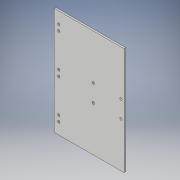
# Autodesk Inventor part: 11 deur plaat
Saved by Autodesk Inventor 2019 (Build 230136000, 136)
## iProperties
Created: 2021-01-22
Part Number: 11 deur plaat
Material: Generic
Document SubType Name: Sheet Metal
Designer: Stefan
Density: 1 g/cm^3
Sheet Metal Rule: Default_mm
Appearance: Default
Author: Stefan
Autodesk Inventor part; units mm, degrees
ref_plane "YZ Plane" through (0, 0, 0) normal (1, 0, 0) x (0, 1, 0)
ref_plane "XZ Plane" through (0, 0, 0) normal (0, 1, 0) x (-1, 0, 0)
ref_plane "XY Plane" through (0, 0, 0) normal (0, 0, 1) x (1, 0, 0)
sketch "Sketch1" plane through (0, 0, 0) normal (0, 0, 1) x (1, 0, 0)
  line L0 (-90.5, -90.5) -> (90.5, -90.5)
  line L1 (90.5, -90.5) -> (90.5, 90.5)
  line L2 (90.5, 90.5) -> (-90.5, 90.5)
  line L3 (-90.5, 90.5) -> (-90.5, -90.5)
  line L4 (-90.5, -90.5) -> (90.5, 90.5) construction
  line L5 (90.5, -90.5) -> (-90.5, 90.5) construction
  point P0 (0, 0)
  dimension "d0" = 181
  dimension "d1" = 181
  constraints: 12 end point, 2 midpoint, 2 parallel, 1 horizontal, 1 perpendicular
  measures "d0" distance of L2.end L1.end
  measures "d1" distance of L1.end L0.end
extrude "Extrusion1" add sketch "Sketch1" along normal blind 3
sketch "Sketch3" plane through (0, 0, 3) normal (0, 0, 1) x (1, 0, 0)
  line L0 (-90.5, 90.5) -> (-90.5, -90.5) projected
  line L1 (-90.5, 82.5) -> (-87.5, 82.5)
  line L2 (-87.5, 82.5) -> (-87.5, 67.5)
  line L3 (-87.5, 67.5) -> (-90.5, 67.5)
  line L4 (-90.5, 67.5) -> (-90.5, 82.5)
  line L5 (-85, 93.5) -> (-90.5, 93.5) projected
  line L6 (-90.5, 52.5) -> (-87.5, 52.5)
  line L7 (-87.5, 52.5) -> (-87.5, 37.5)
  line L8 (-87.5, 37.5) -> (-90.5, 37.5)
  line L9 (-90.5, 37.5) -> (-90.5, 52.5)
  line L10 (-90.5, 22.5) -> (-87.5, 22.5)
  line L11 (-87.5, 22.5) -> (-87.5, 7.5)
  line L12 (-87.5, 7.5) -> (-90.5, 7.5)
  line L13 (-90.5, 7.5) -> (-90.5, 22.5)
  line L14 (-90.5, -7.5) -> (-87.5, -7.5)
  line L15 (-87.5, -7.5) -> (-87.5, -22.5)
  line L16 (-87.5, -22.5) -> (-90.5, -22.5)
  line L17 (-90.5, -22.5) -> (-90.5, -7.5)
  line L18 (-90.5, -37.5) -> (-87.5, -37.5)
  line L19 (-87.5, -37.5) -> (-87.5, -52.5)
  line L20 (-87.5, -52.5) -> (-90.5, -52.5)
  line L21 (-90.5, -52.5) -> (-90.5, -37.5)
  line L22 (-90.5, -67.5) -> (-87.5, -67.5)
  line L23 (-87.5, -67.5) -> (-87.5, -82.5)
  line L24 (-87.5, -82.5) -> (-90.5, -82.5)
  line L25 (-90.5, -82.5) -> (-90.5, -67.5)
  line L26 (87.5, 82.5) -> (90.5, 82.5)
  line L27 (90.5, 82.5) -> (90.5, 67.5)
  line L28 (90.5, 67.5) -> (87.5, 67.5)
  line L29 (87.5, 67.5) -> (87.5, 82.5)
  line L30 (87.5, 52.5) -> (90.5, 52.5)
  line L31 (90.5, 52.5) -> (90.5, 37.5)
  line L32 (90.5, 37.5) -> (87.5, 37.5)
  line L33 (87.5, 37.5) -> (87.5, 52.5)
  line L34 (87.5, 22.5) -> (90.5, 22.5)
  line L35 (90.5, 22.5) -> (90.5, 7.5)
  line L36 (90.5, 7.5) -> (87.5, 7.5)
  line L37 (87.5, 7.5) -> (87.5, 22.5)
  line L38 (87.5, -7.5) -> (90.5, -7.5)
  line L39 (90.5, -7.5) -> (90.5, -22.5)
  line L40 (90.5, -22.5) -> (87.5, -22.5)
  line L41 (87.5, -22.5) -> (87.5, -7.5)
  line L42 (87.5, -37.5) -> (90.5, -37.5)
  line L43 (90.5, -37.5) -> (90.5, -52.5)
  line L44 (90.5, -52.5) -> (87.5, -52.5)
  line L45 (87.5, -52.5) -> (87.5, -37.5)
  line L46 (87.5, -67.5) -> (90.5, -67.5)
  line L47 (90.5, -67.5) -> (90.5, -82.5)
  line L48 (90.5, -82.5) -> (87.5, -82.5)
  line L49 (87.5, -82.5) -> (87.5, -67.5)
  point P0 (0, 0)
  point P1 (-90.5, -93.5)
  dimension "d27" = 3
  dimension "d28" = 15
  dimension "d29" = 11
  dimension "d32" = 30
  dimension "d35" = 178
  constraints: 96 end point, 2 horizontal, 2 parallel, 1 perpendicular, 1 point on line, 1 vertical, 88 other
  measures "d27" distance of L2.end L3.end
  measures "d28" distance of L1.end L2.end
  measures "d29" distance between parallel lines of L5 L1
  measures "d32" distance of L1.start L6.start
  measures "d35" distance of L1.start L26.start
extrude "Extrusion3" cut sketch "Sketch3" against normal blind 3
sketch "Sketch4" plane through (0, 0, 3) normal (0, 0, 1) x (1, 0, 0)
  line L0 (80, 93.5) -> (85.5, 93.5) projected
  line L1 (90.5, 90.5) -> (-90.5, 90.5) projected
  line L2 (85.5, 93.5) -> (90.5, 93.5)
  line L3 (90.5, 93.5) -> (90.5, 90.5)
  line L4 (90.5, 90.5) -> (85.5, 90.5)
  line L5 (85.5, 90.5) -> (85.5, 93.5)
  line L6 (-90.5, -90.5) -> (90.5, -90.5) projected
  line L7 (85.5, -90.5) -> (90.5, -90.5)
  line L8 (90.5, -90.5) -> (90.5, -93.5)
  line L9 (90.5, -93.5) -> (85.5, -93.5)
  line L10 (85.5, -93.5) -> (85.5, -90.5)
  point P0 (0, 0)
  point P1 (85.5, 90.5)
  dimension "d40" = 184
  constraints: 16 end point, 4 parallel, 2 horizontal, 2 perpendicular, 1 point on line
  measures "d40" distance between parallel lines of L1 L9
extrude "Extrusion4" add sketch "Sketch4" against normal blind 3
sketch "Sketch6" plane through (0, 0, 0) normal (0, 0, -1) x (-1, 0, 0)
  line L0 (-90.5, 82.5) -> (-90.5, 93.5) projected
  line L1 (-90.5, 93.5) -> (-75, 93.5)
  line L2 (-75, 93.5) -> (-75, -93.5)
  line L3 (-75, -93.5) -> (-90.5, -93.5)
  line L4 (-90.5, -93.5) -> (-90.5, 93.5)
  line L5 (85, 93.5) -> (90.5, 93.5) projected
  line L6 (90.5, 93.5) -> (46.5, 93.5)
  line L7 (46.5, 93.5) -> (46.5, -93.5)
  line L8 (46.5, -93.5) -> (90.5, -93.5)
  line L9 (90.5, -93.5) -> (90.5, 93.5)
  point P0 (0, 0)
  dimension "d47" = 15.5
  dimension "d48" = 44
  dimension "d49" = 187
  dimension "d50" = 187
  constraints: 16 end point, 4 parallel, 2 horizontal, 2 perpendicular
  measures "d47" distance of L2.end L3.end
  measures "d48" distance of L8.end L7.end
  measures "d49" distance between parallel lines of L5 L3
  measures "d50" distance between parallel lines of L8 L5
extrude "Extrusion6" cut sketch "Sketch6" against normal blind 10
sketch "Sketch7" plane through (0, 0, 3) normal (0, 0, 1) x (1, 0, 0)
  circle A0 centre (-38.5, 73.5) radius 2
  circle A1 centre (-38.5, 63.5) radius 2
  circle A2 centre (-38.5, 5) radius 2
  circle A3 centre (-38.5, -5) radius 2
  circle A4 centre (-38.5, -63.5) radius 2
  circle A5 centre (-38.5, -73.5) radius 2
  line L0 (-40, 93.5) -> (-25, 93.5) projected
  line L1 (-25, -93.5) -> (-40, -93.5) projected
  line L2 (-46.5, 90.5) -> (-46.5, -90.5) projected
  point P0 (0, 0)
  dimension "d53" = 4
  dimension "d54" = 4
  dimension "d55" = 4
  dimension "d56" = 4
  dimension "d57" = 4
  dimension "d58" = 4
  dimension "d59" = 0
  dimension "d60" = 0
  dimension "d61" = 0
  dimension "d62" = 10
  dimension "d63" = 10
  dimension "d64" = 10
  dimension "d65" = 20
  dimension "d66" = 20
  dimension "d67" = 8
  dimension "d68" = 8
  dimension "d69" = 8
  dimension "d70" = 5
  constraints: 6 centre point
  measures "d53" diameter of A0
  measures "d54" diameter of A1
  measures "d55" diameter of A2
  measures "d56" diameter of A3
  measures "d57" diameter of A4
  measures "d58" diameter of A5
  measures "d59" horizontal distance of A1.centre A0.centre
  measures "d60" horizontal distance of A2.centre A3.centre
  measures "d61" horizontal distance of A4.centre A5.centre
  measures "d62" distance of A1.centre A0.centre
  measures "d63" distance of A2.centre A3.centre
  measures "d64" distance of A5.centre A4.centre
  measures "d65" distance from line of L0 A0.centre
  measures "d66" distance from line of L1 A5.centre
  measures "d67" distance from line of L2 A0.centre
  measures "d68" distance from line of L2 A2.centre
  measures "d69" distance from line of A4.centre L2
  measures "d70" vertical distance of point (0, 0) A2.centre
extrude "Extrusion7" cut sketch "Sketch7" against normal blind 10
sketch "Sketch8" plane through (0, 0, 3) normal (0, 0, 1) x (1, 0, 0)
  line L0 (-46.5, 90.5) -> (75, 90.5)
  line L1 (75, 90.5) -> (75, 93.5)
  line L2 (75, 93.5) -> (-46.5, 93.5)
  line L3 (-46.5, 93.5) -> (-46.5, 90.5)
  line L4 (-46.5, -93.5) -> (75, -93.5)
  line L5 (75, -93.5) -> (75, -90.5)
  line L6 (75, -90.5) -> (-46.5, -90.5)
  line L7 (-46.5, -90.5) -> (-46.5, -93.5)
  point P0 (0, 0)
  dimension "d81" = 121.5
  dimension "d82" = 3
  dimension "d85" = 184
  constraints: 16 end point, 2 parallel, 1 collinear, 1 horizontal, 1 perpendicular, 1 vertical, 7 other
  measures "d81" distance of L2.end L1.end
  measures "d82" distance of L1.end L0.end
  measures "d85" distance of L1.end L5.end
extrude "Extrusion8" add sketch "Sketch8" against normal blind 3
sketch "Sketch9" plane through (0, 0, 3) normal (0, 0, 1) x (1, 0, 0)
  line L0 (21.75, 15) -> (69.75, 15) construction
  line L1 (69.75, 15) -> (69.75, -15) construction
  line L2 (69.75, -15) -> (21.75, -15) construction
  line L3 (21.75, -15) -> (21.75, 15) construction
  line L4 (21.75, 15) -> (69.75, -15) construction
  line L5 (69.75, 15) -> (21.75, -15) construction
  line L6 (75, -93.5) -> (75, 93.5) projected
  circle A0 centre (21.75, 15) radius 2
  circle A1 centre (69.75, 15) radius 2
  circle A2 centre (69.75, -15) radius 2
  circle A3 centre (21.75, -15) radius 2
  point P0 (0, 0)
  point P1 (45.75, 0)
  dimension "d92" = 48
  dimension "d93" = 30
  dimension "d94" = 0
  dimension "d95" = 5.25
  dimension "d96" = 4
  dimension "d97" = 4
  dimension "d98" = 4
  dimension "d99" = 4
  constraints: 12 end point, 4 centre point, 4 coincident, 2 midpoint, 2 parallel, 1 horizontal, 1 perpendicular
  measures "d92" distance of L1.end L2.end
  measures "d93" distance of L0.end L1.end
  measures "d94" vertical distance of point (0, 0) point (45.75, 0)
  measures "d95" distance between parallel lines of L6 L1
  measures "d96" diameter of A0
  measures "d97" diameter of A1
  measures "d98" diameter of A2
  measures "d99" diameter of A3
extrude "Extrusion9" cut sketch "Sketch9" against normal blind 3
equation "\"d54\" = d53"
equation "\"d55\" = d53"
equation "\"d56\" = d55"
equation "\"d57\" = d56"
equation "\"d58\" = d57"
equation "\"d63\" = d62"
equation "\"d64\" = d62"
equation "\"d68\" = d67"
equation "\"d69\" = d67"
equation "\"BendRadius\" = Thickness"
equation "\"BendReliefWidth\" = Thickness"
equation "\"BendReliefDepth\" = 0.5 * Thickness"
equation "\"CornerReliefSize\" = 4 * Thickness"
equation "\"MinimumRemnant\" = 2 * Thickness"
equation "\"TransitionRadius\" = BendRadius"
equation "\"JacobiRadiusSize\" = BendRadius"
equation "\"GapSize\" = Thickness"
equation "\"Thickness\" = 0.5"
body "Solid1"
